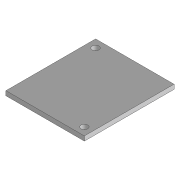
# Autodesk Inventor part: Bottom
Saved by Autodesk Inventor 2022.5 (Build 265521000, 521)
## iProperties
Created: 2020-02-29
Part Number: Bottom
Document SubType Name: Modeling
Designer: Administrator
Density: 1 g/cm^3
Material: Generic
Appearance: Default
Author: Administrator
Autodesk Inventor part; units mm, degrees
ref_plane "YZ Plane" through (0, 0, 0) normal (1, 0, 0) x (0, 1, 0)
ref_plane "XZ Plane" through (0, 0, 0) normal (0, 1, 0) x (-1, 0, 0)
ref_plane "XY Plane" through (0, 0, 0) normal (0, 0, 1) x (1, 0, 0)
sketch "Sketch1" plane through (0, 0, 0) normal (0, 0, 1) x (1, 0, 0)
  line L0 (0, 0) -> (17.5, 0)
  line L1 (17.5, 0) -> (17.5, 20)
  line L2 (17.5, 20) -> (0, 20)
  line L3 (0, 20) -> (0, 0)
  line L4 (0, 0) -> (-17.5, 0)
  line L5 (-17.5, 0) -> (-17.5, -20)
  line L6 (-17.5, -20) -> (0, -20)
  line L7 (0, -20) -> (0, 0)
  line L8 (-17.5, -20) -> (17.5, -20)
  line L9 (17.5, -20) -> (17.5, 20)
  line L10 (17.5, 20) -> (-17.5, 20)
  line L11 (-17.5, 20) -> (-17.5, -20)
  point P0 (0, 20)
  point P1 (0, -20)
  dimension "d7" = 40
  dimension "d8" = 35
  constraints: 24 end point, 6 parallel, 3 horizontal, 3 perpendicular, 2 collinear
  measures "d7" distance of L8.end L1.end
  measures "d8" distance of L1.end L10.end
extrude "Extrusion1" add sketch "Sketch1" along normal blind 2
sketch "Sketch2" plane through (0, 0, 2) normal (0, 0, 1) x (1, 0, 0)
  line L0 (17.5, -20) -> (-17.5, -20) construction
  line L1 (17.5, 20) -> (17.5, -20) construction
  line L2 (-17.5, 20) -> (17.5, 20) construction
  line L3 (-17.5, -20) -> (-17.5, 20) construction
  line L4 (14, 16.5) -> (14, -16.5) construction
  line L5 (14, -16.5) -> (-14, -16.5) construction
  line L6 (-14, -16.5) -> (-14, 16.5) construction
  line L7 (-14, 16.5) -> (14, 16.5) construction
  circle A0 centre (-14, 16.5) radius 1.5
  circle A1 centre (14, -16.5) radius 1.5
  point P0 (0, 0)
  dimension "d9" = 3
  dimension "d10" = 3.5
  constraints: 8 end point, 2 centre point, 2 coincident, 1 equal radius, 3 other
  measures "d9" diameter of A0
  measures "d10" distance between parallel lines of L7 L2
extrude "Extrusion2" cut sketch "Sketch2" against normal through all
body "Solid1"
